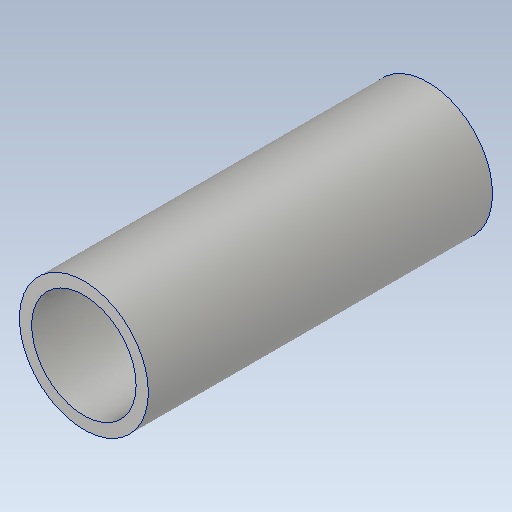
# Autodesk Inventor part: CSP
Saved by Autodesk Inventor 2021 (Build 250183000, 183)
## iProperties
RuleStatus: InUse
Created: 2020-04-27
Part Number: CSP
Material: Aluminium 6082 T6
Document SubType Name: Modeling
Designer: Hannah
Density: 2.7 g/cm^3
Appearance: Aluminum - Flat
Mass: 74.5085 g
Surface Area: 178.606 cm^2
Volume: 27.5957 cm^3
Vendor: Scaffolding Direct
Description: chainstay spacer
Catalog Web Link: https://www.scaffolding-direct.co.uk/5-metre-aluminium-tube-33-7mm-alloy-tube/
length: 90.000 mm
size: 6.000 ul
OD: 33.7
Author: Hannah
Revision Number: 2
Autodesk Inventor part; units mm, degrees
ref_plane "YZ Plane" through (0, 0, 0) normal (1, 0, 0) x (0, 1, 0)
ref_plane "XZ Plane" through (0, 0, 0) normal (0, 1, 0) x (-1, 0, 0)
ref_plane "XY Plane" through (0, 0, 0) normal (0, 0, 1) x (1, 0, 0)
sketch "Sketch1" plane through (0, 0, 0) normal (0, 0, 1) x (1, 0, 0)
  circle A0 centre (0, 0) radius 16.85
  circle A1 centre (0, 0) radius 13.65
  dimension "OD" = 33.7
  dimension "t" = 3.2
  constraints: 2 centre point, 2 coincident
  measures "OD" diameter of A0
  measures "t" radial gap between concentric circles of A0 A1
extrude "Extrusion1" add sketch "Sketch1" along normal mid plane 90
equation "\"size\" = 6"
body "Solid1"
